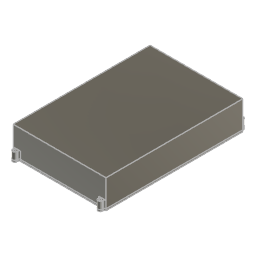
electronics holder (Autodesk Fusion 360 design; units mm, degrees)
part number: 2026-05-19-09-00-51-431
Autodesk Fusion 360 part; units mm, degrees
note: some values were not read from the file. Chosen so that the rebuilt part matches the saved one: which face or edge a step refers to; which pieces of a blend or face edit are solid. Set by a fixed rule: which sketch regions a step uses.
sketch "Sketch3" plane through (0, 0, 0) normal (0, 0, 1) x (1, 0, 0)
  line L0 (5, 13.5) -> (5, -13.5)
  line L1 (5, 13.5) -> (43, 13.5)
  line L2 (43, 13.5) -> (43, -13.5)
  line L3 (43, -13.5) -> (5, -13.5)
  line L4 (5, -13.5) -> (5, 13.5)
  line L5 (-5, -13.5) -> (-43, -13.5)
  line L6 (-43, -13.5) -> (-43, 13.5)
  line L7 (-43, 13.5) -> (-5, 13.5)
  line L8 (-5, 13.5) -> (-5, -13.5)
  line L9 (42.8, 30) -> (-42.8, 30)
  line L10 (42.8, 30) -> (-42.8, 30)
  line L11 (-42.8, 30) -> (-42.8, 86.5)
  line L12 (-42.8, 86.5) -> (42.8, 86.5)
  line L13 (42.8, 86.5) -> (42.8, 30)
  point P0 (5, 0)
  point P1 (0, 30)
  dimension "d5" = 27
  dimension "d6" = 38
  dimension "d7" = 27
  dimension "d8" = 38
  dimension "d9" = 27
  dimension "d10" = 85.6
  dimension "d11" = 56.5
  constraint midpoint L0 P0
  constraint vertical L0
  constraint horizontal L1
  constraint vertical L2
  constraint horizontal L3
  constraint vertical L4
  constraint horizontal L5
  constraint vertical L6
  constraint horizontal L7
  constraint vertical L8
  constraint midpoint L9 P1
  constraint horizontal L9
  constraint horizontal L10
  constraint vertical L11
  constraint horizontal L12
  constraint vertical L13
  measures "d5" distance of L0.start L0.end
  measures "d6" distance of L0.start L1.end
  measures "d7" distance of L0.start L0.end
  measures "d8" distance of L5.start L5.end
  measures "d9" distance of L5.start L7.end
  measures "d10" distance of L9.start L9.end
  measures "d11" distance of L9.start L12.end
extrude "Extrude2" add sketch "Sketch3" along normal blind 18 makes body 1 at (-30.3333, -4.5, 0) makes body 2 at (17.6667, -4.5, 0) makes body 3 at (14.2667, 48.8333, 0)
sketch "Sketch4" plane through (0, 0, 0) normal (0, 0, -1) x (1, 0, 0)
  line L0 (-42.8, -86.5) -> (42.8, -86.5)
  line L1 (42.8, -86.5) -> (42.8, -30)
  line L2 (42.8, -30) -> (-42.8, -30)
  line L3 (-42.8, -30) -> (-42.8, -86.5)
  line L4 (-52.8376, 24.1534) -> (52.8376, 24.1534)
  line L5 (52.8376, 24.1534) -> (52.8376, -104.1534)
  line L6 (52.8376, -104.1534) -> (-52.8376, -104.1534)
  line L7 (-52.8376, -104.1534) -> (-52.8376, 24.1534)
  line L8 (-52.8376, 24.1534) -> (52.8376, -104.1534) construction
  line L9 (52.8376, 24.1534) -> (-52.8376, -104.1534) construction
  line L10 (-76.82, -19.5117) -> (-61.32, -19.5117)
  line L11 (-61.32, -19.5117) -> (-61.32, 0.8883)
  line L12 (-61.32, 0.8883) -> (-76.82, 0.8883)
  line L13 (-76.82, 0.8883) -> (-76.82, -19.5117)
  point P0 (0, -40)
  dimension "d16" = 15.5
  dimension "d17" = 20.4
  constraint horizontal L4
  constraint perpendicular L4 L5
  constraint parallel L4 L6
  constraint parallel L5 L7
  constraint coincident L8 P0
  constraint coincident L9 P0
  constraint horizontal L10
  constraint vertical L11
  constraint horizontal L12
  constraint vertical L13
  measures "d16" distance of L10.start L10.end
  measures "d17" distance of L10.start L12.end
extrude "Extrude3" add sketch "Sketch4" along normal blind 2 separate body contours L0 L1 L2 L3 | L4 L5 L6 L7 makes body 4
extrude "Extrude4" add 1 faces at (52.8376, 18.6155, -0.6667) along direction (1, 0, 0) blind 20 on bodies 4 bodies 4
sketch "Sketch5" plane through (0, 0, 0) normal (0, 0, 1) x (-1, 0, 0)
  line L0 (-72.8376, -104.1534) -> (52.8376, -104.1534)
  line L1 (52.8376, -104.1534) -> (52.8376, 24.1534)
  line L2 (52.8376, 24.1534) -> (-72.8376, 24.1534)
  line L3 (-72.8376, 24.1534) -> (-72.8376, -104.1534)
  line L4 (-50, 10) -> (-65.5, 10)
  line L5 (-65.5, 10) -> (-65.5, -10.4)
  line L6 (-65.5, -10.4) -> (-50, -10.4)
  line L7 (-50, -10.4) -> (-50, 10)
  dimension "d20" = 15.5
  dimension "d21" = 20.4
  constraint horizontal L4
  constraint vertical L5
  constraint horizontal L6
  constraint vertical L7
  measures "d20" distance of L4.start L4.end
  measures "d21" distance of L4.start L6.end
extrude "Extrude5" add sketch "Sketch5" along normal blind 11 separate body contours L4 L5 L6 L7 makes body 5
extrude "Extrude6" add 1 faces at (72.8376, 18.6155, -0.6667) along direction (1, 0, 0) blind 2 on bodies 4 bodies 4
move_body "Move4" bodies 3 to x (1, 0, 0) y (0, 1, 0) z (0, 0, 1) at (0, -10, 0)
extrude "Extrude7" add 1 faces at (-10.2792, -24.1534, -0.6667) along direction (0, -1, 0) blind 60 on bodies 4 bodies 4
sketch "Sketch6" plane through (0, 0, 0) normal (0, 0, 1) x (-1, 0, 0)
  line L0 (-74.8376, -104.1534) -> (52.8376, -104.1534)
  line L1 (52.8376, -104.1534) -> (52.8376, 84.1534)
  line L2 (52.8376, 84.1534) -> (-74.8376, 84.1534)
  line L3 (-74.8376, 84.1534) -> (-74.8376, -104.1534)
  line L4 (-55.6225, 66.6829) -> (-1.6225, 66.6829)
  line L5 (-1.6225, 66.6829) -> (-1.6225, 7.1829)
  line L6 (-1.6225, 7.1829) -> (-55.6225, 7.1829)
  line L7 (-55.6225, 7.1829) -> (-55.6225, 66.6829)
  dimension "d28" = 54
  dimension "d29" = 59.5
  constraint horizontal L4
  constraint vertical L5
  constraint horizontal L6
  constraint vertical L7
  measures "d28" distance of L4.start L4.end
  measures "d29" distance of L4.start L6.end
extrude "Extrude8" add sketch "Sketch6" along normal blind 27.5 separate body contours L4 L5 L6 L7 makes body 6
move_body "Move5" bodies 6 to x (1, 0, 0) y (0, 1, 0) z (0, 0, 1) at (10, -13, 0)
copy_body "CopyPasteBodies5" bodies 6 makes body 7
move_body "Move7" bodies 7 to x (1, 0, 0) y (0, 1, 0) z (0, 0, 1) at (-55, 0, 0)
extrude "Extrude10" add 1 faces at (-10.2792, -84.1534, -0.6667) along direction (0, -1, 0) blind 5 on bodies 4 bodies 4
extrude "Extrude11" add 1 faces at (-10.2792, 104.1534, -0.6667) along direction (0, 1, 0) blind 30 on bodies 4 bodies 4
move_body "Move8" bodies 3 to x (0, -1, 0) y (1, 0, 0) z (0, 0, 1) at (-34.5302, 62.1751, 0)
move_body "Move9" bodies 1 to x (0, -1, 0) y (1, 0, 0) z (0, 0, 1) at (-32.393, -21.4631, 0)
move_body "Move10" bodies 2 to x (0, -1, 0) y (1, 0, 0) z (0, 0, 1) at (-31.9661, 67.0384, 0)
move_body "Move11" bodies 3 to x (1, 0, 0) y (0, 1, 0) z (0, 0, 1) at (2.2501, -30.8582, 0)
move_body "Move12" bodies 2 to x (1, 0, 0) y (0, 1, 0) z (0, 0, 1) at (-1.6072, 11.8933, 0)
move_body "Move13" bodies 1 to x (1, 0, 0) y (0, 1, 0) z (0, 0, 1) at (-0.6429, 5.143, 0)
extrude "Extrude12" cut 1 faces at (-10.2792, 134.1534, -0.6667) along direction (0, -1, 0) blind 15 on bodies 4 bodies 4
move_body "Move14" bodies 5 to x (0, -1, 0) y (1, 0, 0) z (0, 0, 1) at (60, 40, 0)
move_body "Move15" bodies 5 to x (1, 0, 0) y (0, 1, 0) z (0, 0, 1) at (-1.4153, 18.1129, 0)
copy_body "CopyPasteBodies6" bodies 5 makes body 8
move_body "Move16" bodies 8 to x (1, 0, 0) y (0, 1, 0) z (0, 0, 1) at (0, 20, 0)
copy_body "CopyPasteBodies7" bodies 8 makes body 9
move_body "Move17" bodies 9 to x (1, 0, 0) y (0, 1, 0) z (0, 0, 1) at (0, 20, 0)
sketch "Sketch7" plane through (0, 0, 0) normal (0, 0, 1) x (-1, 0, 0)
  line L0 (-74.8376, -119.1534) -> (52.8376, -119.1534)
  line L1 (52.8376, -119.1534) -> (52.8376, 89.1534)
  line L2 (52.8376, 89.1534) -> (-74.8376, 89.1534)
  line L3 (-74.8376, 89.1534) -> (-74.8376, -119.1534)
  line L4 (-68.8465, -53.2998) -> (-53.3465, -53.2998)
  line L5 (-53.3465, -53.2998) -> (-53.3465, -79.0998)
  line L6 (-53.3465, -79.0998) -> (-68.8465, -79.0998)
  line L7 (-68.8465, -79.0998) -> (-68.8465, -53.2998)
  dimension "d40" = 15.5
  dimension "d41" = 25.8
  constraint horizontal L4
  constraint vertical L5
  constraint horizontal L6
  constraint vertical L7
  measures "d40" distance of L4.start L4.end
  measures "d41" distance of L4.start L6.end
extrude "Extrude13" add sketch "Sketch7" along normal blind 3 separate body contours L4 L5 L6 L7 makes body 10
extrude "Extrude14" cut 1 faces at (-10.2792, 119.1534, -0.6667) along direction (0, -1, 0) blind 20 on bodies 4 bodies 4
move_body "Move18" bodies 3 to x (1, 0, 0) y (0, 1, 0) z (0, 0, 1) at (0, -5, 0)
sketch "Sketch8" plane through (0, 0, 0) normal (0, 0, 1) x (-1, 0, 0)
  line L0 (-74.8376, -99.1534) -> (52.8376, -99.1534)
  line L1 (52.8376, -99.1534) -> (52.8376, 89.1534)
  line L2 (52.8376, 89.1534) -> (-74.8376, 89.1534)
  line L3 (-74.8376, 89.1534) -> (-74.8376, -99.1534)
  line L4 (-74.8376, 89.1534) -> (-69.8376, 89.1534)
  line L5 (-69.8376, 89.1534) -> (-69.8376, 92.1534)
  circle A0 centre (-69.8376, 92.1534) radius 1.5
  line L6 (52.8376, 89.1534) -> (47.8376, 89.1534)
  line L7 (47.8376, 89.1534) -> (47.8376, 92.1534)
  circle A1 centre (47.8376, 92.1534) radius 1.5
  circle A2 centre (47.8376, 92.1534) radius 3
  circle A3 centre (-69.8376, 92.1534) radius 3
  line L8 (-69.8376, 92.1534) -> (-72.8376, 92.1534)
  line L9 (-72.8376, 92.1534) -> (-72.8376, 89.1533)
  line L10 (-66.8376, 92.1534) -> (-66.8376, 89.1534)
  line L11 (-66.8376, 89.1534) -> (-69.8376, 89.1534)
  line L12 (47.8376, 92.1534) -> (44.8376, 92.1534)
  line L13 (44.8376, 92.1534) -> (44.8376, 89.1534)
  line L14 (50.8376, 92.1534) -> (50.8376, 89.2905)
  line L15 (50.8376, 89.2905) -> (50.8376, 89.2)
  line L16 (50.8376, 89.2) -> (50.8398, 89.1534)
  line L17 (-11, 89.1534) -> (-11, -99.1534)
  line L18 (-11, -5) -> (37.3566, -5)
  circle A4 centre (-69.8376, -102.1534) radius 3
  line L19 (-69.8376, -102.1534) -> (-72.8376, -102.1534)
  line L20 (-72.8376, -102.1534) -> (-72.8376, -99.1533)
  line L21 (-74.8376, -99.1534) -> (-74.8376, 89.1534)
  line L22 (52.8376, -99.1534) -> (-74.8376, -99.1534)
  line L23 (-74.8376, -99.1534) -> (-69.8376, -99.1534)
  circle A5 centre (-69.8376, -102.1534) radius 1.5
  line L24 (-69.8376, -99.1534) -> (-69.8376, -102.1534)
  line L25 (-66.8376, -102.1534) -> (-66.8376, -99.1534)
  circle A6 centre (47.8376, -102.1534) radius 3
  circle A7 centre (47.8376, -102.1534) radius 1.5
  line L26 (52.8376, 89.1534) -> (52.8376, -99.1534)
  line L27 (52.8376, -99.1534) -> (47.8376, -99.1534)
  line L28 (50.8376, -102.1534) -> (50.8376, -99.2905)
  line L29 (47.8376, -102.1534) -> (44.8376, -102.1534)
  line L30 (44.8376, -102.1534) -> (44.8376, -99.1534)
  line L31 (47.8376, -99.1534) -> (47.8376, -102.1534)
  line L32 (50.8376, -99.2905) -> (50.8376, -99.2)
  line L33 (50.8398, -99.1534) -> (47.8376, -99.1534)
  line L34 (50.8376, -99.2) -> (50.8398, -99.1534)
  point P0 (50.8398, -99.1534)
  dimension "d46" = 5
  dimension "d47" = 3
  dimension "d48" = 3
  dimension "d49" = 5
  dimension "d50" = 3
  dimension "d51" = 3
  dimension "d52" = 6
  dimension "d53" = 6
  dimension "d54" = 90
  constraint coincident L2.end L3.start
  constraint perpendicular L3 L4
  constraint perpendicular L4 L5
  constraint coincident L5.end A0.centre
  constraint coincident L1.end L2.start
  constraint perpendicular L1 L6
  constraint perpendicular L6 L7
  constraint coincident L7.end A1.centre
  constraint concentric A1 A2
  constraint concentric A0 A3
  constraint coincident A3 L8.end
  constraint perpendicular L5 L8
  constraint coincident A3 L10.start
  constraint coincident L2 L10.end
  constraint tangent A3 L10
  constraint perpendicular L2 L10
  constraint coincident A2 L12.end
  constraint perpendicular L7 L12
  constraint coincident L2 L13.end
  constraint tangent A2 L13
  constraint coincident A2 L14.start
  constraint tangent A2 L14
  constraint perpendicular L6 L14
  constraint perpendicular L6 L15
  constraint coincident L6 L16.end
  constraint midpoint L2 L17.start
  constraint midpoint L0 L17.end
  constraint midpoint L17 L18.start
  constraint perpendicular L17 L18
  constraint symmetric L0.start L18 L2.end
  constraint symmetric L0.end L18 L1.end
  constraint symmetric L1.end L18 L0.end
  constraint symmetric L2.end L18 L0.start
  constraint symmetric L4.end L18 L23.end
  constraint symmetric L5.end L18 A4.centre
  constraint symmetric A0 L18 A5
  constraint symmetric L6.end L18 L27.end
  constraint symmetric L7.end L18 A6.centre
  constraint symmetric A1 L18 A7
  constraint symmetric A2 L18 A6
  constraint symmetric A3 L18 A4
  constraint symmetric L8.end L18 L19.end
  constraint symmetric L9.end L18 L20.end
  constraint symmetric L10.start L18 L25.start
  constraint symmetric L10.end L18 L25.end
  constraint symmetric L12.end L18 L29.end
  constraint symmetric L13.end L18 L30.end
  constraint symmetric L14.start L18 L28.start
  constraint symmetric L14.end L18 L28.end
  constraint symmetric L15.end L18 L32.end
  constraint symmetric L16.end L18 P0
  constraint coincident P0 L33.start
  measures "d46" distance of L2.end L4.end
  measures "d47" distance of L4.end L5.end
  measures "d48" diameter of A0
  measures "d49" distance of L1.end L6.end
  measures "d50" distance of L6.end L7.end
  measures "d51" diameter of A1
  measures "d52" diameter of A2
  measures "d53" diameter of A3
  measures "d54" angle of L8 L9
extrude "Extrude15" add sketch "Sketch8" against normal blind 2.4 contours L0 A4 L20 L22 L23 | L0 A4 L22 L25 | A4 L19 A5 L24 | A4 L19 A5 L24 | L2 L4 A3 L9 | L2 A3 L10 L11 | L5 A0 A3 L8 | L5 A0 A3 L8 | L0 L22 A6 L30 | L0 L22 A6 L27 L28 L32 L33 L34 | A6 A7 L29 L31 | A6 A7 L29 L31 | L2 A2 L13 | L2 L6 A2 L14 L15 L16 | L7 A1 A2 L12 | L7 A1 A2 L12 bodies 4
extrude "Extrude16" add 1 faces at (29.6125, 36.3845, -2) along direction (0, 0, -1) blind 0.4 on bodies 4 bodies 4
fillet "Fillet1" radius 2 1 edges at (72.8376, -89.1534, -1.2) on bodies 4
fillet "Fillet2" radius 2 1 edges at (66.8376, -89.1534, -1.2) on bodies 4
fillet "Fillet3" radius 2 6 edges at (-50.8376, -89.2, -1.2) (-44.8376, -89.1534, -1.2) (72.8376, 99.1534, -1.2) (66.8376, 99.1534, -1.2) (-50.8376, 99.2, -1.2) (-44.8376, 99.1534, -1.2) on bodies 4
fillet "Fillet4" radius 2 1 edges at (-50.8398, -89.1534, -1.2) on bodies 4
sketch "Sketch9" plane through (0, 0, 0) normal (0, 0, 1) x (-1, 0, 0)
  circle A0 centre (-69.8376, 92.1534) radius 1.5
  circle A1 centre (47.8376, -102.1534) radius 1.5
  circle A2 centre (47.8376, 92.1534) radius 1.5
  circle A3 centre (-69.8376, -102.1534) radius 1.5
  arc A4 (-72.8376, -101.1534) -> (-74.8376, -99.1534) centre (-74.8376, -101.1534) ccw
  line L0 (-72.8376, -101.1534) -> (-72.8376, -102.1534)
  arc A5 (-72.8376, -102.1534) -> (-66.8376, -102.1534) centre (-69.8376, -102.1534) ccw
  line L1 (-66.8376, -102.1534) -> (-66.8376, -101.1534)
  arc A6 (-64.8376, -99.1534) -> (-66.8376, -101.1534) centre (-64.8376, -101.1534) ccw
  line L2 (-64.8376, -99.1534) -> (42.8376, -99.1534)
  arc A7 (44.8376, -101.1534) -> (42.8376, -99.1534) centre (42.8376, -101.1534) ccw
  line L3 (44.8376, -101.1534) -> (44.8376, -102.1534)
  arc A8 (44.8376, -102.1534) -> (50.8376, -102.1534) centre (47.8376, -102.1534) ccw
  line L4 (50.8376, -102.1534) -> (50.8376, -99.2475)
  arc A9 (50.8398, -99.1534) -> (50.8376, -99.2475) centre (52.8376, -99.2475) ccw
  line L5 (50.8398, -99.1534) -> (52.8376, -99.1534)
  line L6 (52.8376, -99.1534) -> (52.8376, 89.1534)
  arc A10 (50.8376, 91.1534) -> (52.8376, 89.1534) centre (52.8376, 91.1534) ccw
  line L7 (50.8376, 91.1534) -> (50.8376, 92.1534)
  arc A11 (50.8376, 92.1534) -> (44.8376, 92.1534) centre (47.8376, 92.1534) ccw
  line L8 (44.8376, 92.1534) -> (44.8376, 91.1534)
  arc A12 (42.8376, 89.1534) -> (44.8376, 91.1534) centre (42.8376, 91.1534) ccw
  line L9 (42.8376, 89.1534) -> (-64.8376, 89.1534)
  arc A13 (-66.8376, 91.1534) -> (-64.8376, 89.1534) centre (-64.8376, 91.1534) ccw
  line L10 (-66.8376, 91.1534) -> (-66.8376, 92.1534)
  arc A14 (-66.8376, 92.1534) -> (-72.8376, 92.1534) centre (-69.8376, 92.1534) ccw
  line L11 (-72.8376, 92.1534) -> (-72.8376, 91.1534)
  arc A15 (-74.8376, 89.1534) -> (-72.8376, 91.1534) centre (-74.8376, 91.1534) ccw
  line L12 (-74.8376, 89.1534) -> (-74.8376, -99.1534)
  line L13 (52.8376, -99.1534) -> (52.8398, -99.1534)
  line L14 (50.8398, -101.1534) -> (50.8398, -103.2837)
  line L15 (52.8376, -99.1534) -> (52.8376, -102)
  line L16 (52.8376, -102) -> (50.8398, -102)
  arc A16 (52.8398, -99.1534) -> (50.8398, -101.1534) centre (52.8398, -101.1534) ccw
  line L17 (50.9, -102) -> (50.3077, -100.0414)
  line L18 (50.3077, -100.0414) -> (50.5604, -98.5323)
  line L19 (50.5604, -98.5323) -> (52.8398, -99.1534)
  dimension "d67" = 2
  constraint coincident L5.end L6.start
  constraint vertical L14
  constraint perpendicular L5 L15
  constraint coincident L14 L16.end
  constraint perpendicular L4 L16
  constraint tangent L13 A16
  constraint tangent L14 A16
  constraint coincident L16 L17.start
  measures "d67" radius of A16
extrude "Extrude17" add sketch "Sketch9" against normal blind 2.4 contours L4 A9 L5 L14 L17 L18 L19 | L4 A9 L5 A16 bodies 4
sketch "Sketch10" plane through (0, 0, 0) normal (0, 0, 1) x (-1, 0, 0)
  line L0 (50.8376, -101.801) -> (50.8376, -101.1534)
  arc A0 (52.8376, -99.1534) -> (50.8398, -101.1534) centre (52.8398, -101.1534) ccw
  line L1 (52.8376, -99.1534) -> (52.8376, 89.1534)
  arc A1 (50.8376, 91.1534) -> (52.8376, 89.1534) centre (52.8376, 91.1534) ccw
  line L2 (50.8376, 91.1534) -> (50.8376, 92.1534)
  arc A2 (50.8376, 92.1534) -> (44.8376, 92.1534) centre (47.8376, 92.1534) ccw
  line L3 (44.8376, 92.1534) -> (44.8376, 91.1534)
  arc A3 (42.8376, 89.1534) -> (44.8376, 91.1534) centre (42.8376, 91.1534) ccw
  line L4 (42.8376, 89.1534) -> (-64.8376, 89.1534)
  arc A4 (-66.8376, 91.1534) -> (-64.8376, 89.1534) centre (-64.8376, 91.1534) ccw
  line L5 (-66.8376, 91.1534) -> (-66.8376, 92.1534)
  arc A5 (-66.8376, 92.1534) -> (-72.8376, 92.1534) centre (-69.8376, 92.1534) ccw
  line L6 (-72.8376, 92.1534) -> (-72.8376, 91.1534)
  arc A6 (-74.8376, 89.1534) -> (-72.8376, 91.1534) centre (-74.8376, 91.1534) ccw
  line L7 (-74.8376, 89.1534) -> (-74.8376, -99.1534)
  arc A7 (-72.8376, -101.1534) -> (-74.8376, -99.1534) centre (-74.8376, -101.1534) ccw
  line L8 (-72.8376, -101.1534) -> (-72.8376, -102.1534)
  arc A8 (-72.8376, -102.1534) -> (-66.8376, -102.1534) centre (-69.8376, -102.1534) ccw
  line L9 (-66.8376, -102.1534) -> (-66.8376, -101.1534)
  arc A9 (-64.8376, -99.1534) -> (-66.8376, -101.1534) centre (-64.8376, -101.1534) ccw
  line L10 (-64.8376, -99.1534) -> (42.8376, -99.1534)
  arc A10 (44.8376, -101.1534) -> (42.8376, -99.1534) centre (42.8376, -101.1534) ccw
  line L11 (44.8376, -101.1534) -> (44.8376, -102.1534)
  arc A11 (44.8376, -102.1534) -> (50.8376, -102.1534) centre (47.8376, -102.1534) ccw
  line L12 (50.8376, -102.1534) -> (50.8376, -101.801)
  circle A12 centre (-69.8376, -102.1534) radius 1.5
  circle A13 centre (47.8376, 92.1534) radius 1.5
  circle A14 centre (47.8376, -102.1534) radius 1.5
  circle A15 centre (-69.8376, 92.1534) radius 1.5
  line L13 (-74.8376, -99.1534) -> (-74.8376, -97.1534)
  line L14 (-74.8376, -99.1534) -> (-72.8376, -99.1534)
  line L15 (-72.8376, -99.1534) -> (-73.0068, 88.2092)
  line L16 (-74.8376, 89.1534) -> (-74.8376, 87.1534)
  line L17 (-74.8376, 87.1534) -> (52.7862, 87.1534)
  line L18 (52.8376, 89.1534) -> (50.8376, 89.1534)
  line L19 (50.8376, 89.1534) -> (50.8376, -98)
  line L20 (52.8376, -99.1534) -> (52.8376, -97.1534)
  line L21 (52.8376, -97.1534) -> (-74.8376, -97.1534)
  line L22 (52.8376, -97.1534) -> (52.8376, 89.1534)
  line L23 (-74.8376, -97.1534) -> (52.8376, -97.1534)
  arc A16 (44.8376, -102.1534) -> (50.8376, -102.1534) centre (47.8376, -102.1534) ccw
  arc A17 (52.8376, -99.1534) -> (50.8398, -101.1534) centre (52.8398, -101.1534) ccw
  line L24 (50.8387, -101.801) -> (50.8387, -101.1534)
  line L25 (50.8376, -102.1534) -> (50.8387, -101.801)
  line L26 (44.8376, -102.1534) -> (44.8376, -101.1534)
  arc A18 (44.8376, -101.1534) -> (42.8376, -99.1534) centre (42.8376, -101.1534) ccw
  line L27 (-64.8376, -99.1534) -> (42.8376, -99.1534)
  arc A19 (-72.8376, -101.1534) -> (-74.8376, -99.1534) centre (-74.8376, -101.1534) ccw
  arc A20 (-72.8376, -102.1534) -> (-66.8376, -102.1534) centre (-69.8376, -102.1534) ccw
  line L28 (-72.8376, -102.1534) -> (-72.8376, -101.1534)
  line L29 (-66.8376, -102.1534) -> (-66.8376, -101.1534)
  arc A21 (-64.8376, -99.1534) -> (-66.8376, -101.1534) centre (-64.8376, -101.1534) ccw
  line L30 (47.8376, -99.1534) -> (47.8376, -102.1534)
  circle A22 centre (47.8376, -102.1534) radius 3
  line L31 (47.8376, -102.1534) -> (44.8376, -102.1534)
  circle A23 centre (47.8376, -102.1534) radius 1.5
  circle A24 centre (-69.8376, -102.1534) radius 3
  line L32 (-66.8376, -102.1534) -> (-66.8376, -99.1534)
  circle A25 centre (-69.8376, -102.1534) radius 1.5
  line L33 (-69.8376, -102.1534) -> (-72.8376, -102.1534)
  line L34 (-69.8376, -99.1534) -> (-69.8376, -102.1534)
  line L35 (-72.8376, -102.1534) -> (-72.8376, -99.1533)
  line L36 (50.8376, -102.1534) -> (50.8376, -101.1534)
  line L37 (50.8387, -101.1534) -> (52.8376, -99.1534)
  arc A26 (52.8376, -99.1534) -> (50.8376, -101.1534) centre (52.8376, -101.1534) ccw
  line L38 (52.8376, -99.1534) -> (-74.8376, -99.1534)
  line L39 (-74.8376, 89.1534) -> (52.8376, 89.1534)
  point P0 (-66.8376, -101.1534)
  point P1 (50.8376, -99.1534)
  dimension "d70" = 2
  dimension "d71" = 2
  dimension "d72" = 2
  dimension "d73" = 90
  dimension "d74" = 2
  dimension "d75" = 2
  dimension "d76" = 3
  dimension "d77" = 2
  constraint coincident L7.end A7.end
  constraint parallel L7 L13
  constraint perpendicular L7 L14
  constraint coincident A6.start L7.start
  constraint parallel L7 L16
  constraint coincident L1.end A1.end
  constraint tangent A1 L18
  constraint perpendicular L10 L19
  constraint coincident A0.start L1.start
  constraint coincident L1 L20.end
  constraint vertical L36
  constraint coincident A11.end L12.start
  constraint coincident L24.end L37.start
  constraint coincident P1 L36
  constraint tangent L36 A26
  measures "d70" distance of L7.end L13.end
  measures "d71" distance of L7.end L14.end
  measures "d72" distance of A6.start L16.end
  measures "d73" angle of L16 L17
  measures "d74" distance of L1.end L18.end
  measures "d75" distance of A0.start L20.end
  measures "d76" distance of A11.end P1
  measures "d77" radius of A26
extrude "Extrude18" add sketch "Sketch10" along normal blind 50 separate body contours L0 A0 L12 A17 L24 L25 A22 L36 A26 L38 | A11 A14 A16 L30 A22 L31 A23 | L1 L10 L15 L20 L21 L23 L27 L38 | A10 L11 L26 A18 A22 L38 | A14 L30 A22 L31 A23 | L1 L18 L19 L21 L22 L23 L39 | A1 L2 A2 L3 A3 L18 L39 | A9 A21 L32 L38 | L4 L7 L16 L17 L19 L39 | L7 L15 L17 L21 L23 | L7 L13 L14 L15 L21 L23 L38 | L9 L29 A24 L32 L38 | A7 L14 A19 L35 L38 | L8 L28 A24 L35 L38 | A8 A12 A20 A24 A25 L33 L34 | A12 A24 A25 L33 L34 | A4 L5 A5 L6 A6 L39 makes body 11
extrude "Extrude19" cut 1 faces at (-47.4321, -89.1566, 50) along direction (0, 0, -1) blind 40 on bodies 11 bodies 11
extrude "Extrude20" add sketch "Sketch10" along normal blind 30 separate body contours L1 L10 L15 L20 L21 L23 L27 L38 | L1 L18 L19 L21 L22 L23 L39 | L4 L7 L16 L17 L19 L39 | L7 L15 L17 L21 L23 | L7 L13 L14 L15 L21 L23 L38 makes body 12
combine "Combine1" operation add target body 12 tool bodies 11
move_face "OffsetFaces1" offset 0.168 1 faces at (72.8949, 35.7178, 10) on bodies 12
extrude "Extrude21" add 1 faces at (-7.0013, 97.82, 30) along direction (0, 0, 1) blind 5 on bodies 12 bodies 12
sketch "Sketch11" plane through (0, 0, 35) normal (0, 0, 1) x (-1, 0, 0)
  line L0 (50.8376, -97.1534) -> (-72.6714, -97.1534)
  line L1 (-72.6714, -97.1534) -> (-72.8379, 87.1534)
  line L2 (-72.8379, 87.1534) -> (50.8376, 87.1534)
  line L3 (50.8376, 87.1534) -> (50.8376, -97.1534)
  line L4 (-74.8376, 89.1534) -> (-74.8376, -99.1534)
  line L5 (-74.8376, -99.1534) -> (52.8376, -99.1534)
  line L6 (52.8376, -99.1534) -> (52.8376, 89.1534)
  line L7 (52.8376, 89.1534) -> (-74.8376, 89.1534)
  line L8 (-74.8376, 89.1534) -> (52.8376, 89.1534)
  line L9 (52.8376, 89.1534) -> (52.8376, -99.1534)
  line L10 (52.8376, -99.1534) -> (-74.8376, -99.1534)
  line L11 (-74.8376, -99.1534) -> (-74.8376, 89.1534)
  constraint horizontal L8
  constraint vertical L9
  constraint horizontal L10
  constraint vertical L11
  constraint coincident L5.end L6.start
  constraint coincident L4.start L7.end
extrude "Extrude22" add sketch "Sketch11" along normal blind 2 contours L0 L1 L2 L3 | L4 L5 L6 L7 L8 L9 L10 L11 bodies 12
sketch "Sketch12" plane through (74.8376, 0, 0) normal (1, 0, 0) x (0, 1, 0)
  line L0 (99.1534, 10) -> (99.1534, 35)
  line L1 (99.1534, 35) -> (99.1534, 37)
  line L2 (99.1534, 37) -> (-89.1534, 37)
  line L3 (-89.1534, 37) -> (-89.1534, 10)
  line L4 (-89.1534, 10) -> (-89.1534, 0)
  line L5 (-89.1534, 0) -> (99.1534, 0)
  line L6 (99.1534, 0) -> (99.1534, 10)
  line L7 (5, 37) -> (5, -2.4)
  line L8 (5, 17.3) -> (5, 26.825)
  line L9 (5, 17.3) -> (5, 7.775)
  line L10 (5, 7.775) -> (14.525, 7.775)
  line L11 (14.525, 7.775) -> (14.525, 26.825)
  line L12 (14.525, 26.825) -> (-4.525, 26.825)
  line L13 (-4.525, 26.825) -> (-4.525, 7.775)
  line L14 (-4.525, 7.775) -> (14.525, 7.775)
  point P0 (5, 26.1052)
  dimension "d90" = 9.525
  dimension "d91" = 9.525
  dimension "d92" = 9.525
  dimension "d93" = 19.05
  dimension "d94" = 19.05
  dimension "d95" = 19.05
  constraint midpoint L2 L7.start
  constraint perpendicular L5 L7
  constraint midpoint L7 L8.start
  constraint parallel L7 L8
  constraint parallel L7 L9
  constraint perpendicular L7 L10
  constraint perpendicular L10 L11
  constraint perpendicular L7 L12
  constraint perpendicular L12 L13
  measures "d90" distance of L8.start L8.end
  measures "d91" distance of L8.start L9.end
  measures "d92" distance of L9.end L10.end
  measures "d93" distance of L10.end L11.end
  measures "d94" distance of L11.end L12.end
  measures "d95" distance of L12.end L13.end
sketch "Sketch13" plane through (0, 0, 37) normal (0, 0, 1) x (-1, 0, 0)
  line L0 (-74.8376, -99.1534) -> (52.8376, -99.1534)
  line L1 (52.8376, -99.1534) -> (52.8376, 89.1534)
  line L2 (52.8376, 89.1534) -> (-74.8376, 89.1534)
  line L3 (-74.8376, 89.1534) -> (-74.8376, -99.1534)
  circle A0 centre (154.6142, -13.5152) radius 4.572
  circle A1 centre (154.6142, -13.5152) radius 5
  dimension "d96" = 9.144
  dimension "d97" = 10
  constraint concentric A0 A1
  measures "d96" diameter of A0
  measures "d97" diameter of A1
combine "Combine2" [no effect]
sketch "Sketch14" plane through (0, 0, 0) normal (1, 0, 0) x (0, 1, 0)
  circle A0 centre (-180, 10) radius 4
  circle A1 centre (-180, 10) radius 7.5
  dimension "d102" = 8
  dimension "d103" = 15
  constraint concentric A0 A1
  measures "d102" diameter of A0
  measures "d103" diameter of A1
extrude "Extrude25" add sketch "Sketch14" along normal blind 2 separate body makes body 13
sketch "Sketch15" plane through (2, 0, 0) normal (1, 0, 0) x (0, 1, 0)
  circle A0 centre (-180, 10) radius 4
  circle A1 centre (-180, 10) radius 7.5
  circle A2 centre (-180, 10) radius 5
  circle A3 centre (-180, 10) radius 10
  dimension "d106" = 10
  dimension "d107" = 20
  constraint concentric A0 A2
  constraint concentric A0 A3
  measures "d106" diameter of A2
  measures "d107" diameter of A3
extrude "Extrude26" add sketch "Sketch15" along normal blind 3 contours A1 | A3 bodies 13
extrude "Extrude27" add 1 faces at (2, -170.8985, 9.1306) along direction (-1, 0, 0) blind 2 on bodies 13 bodies 13
sketch "Sketch16" plane through (0, 0, 0) normal (-1, 0, 0) x (0, -1, 0)
  circle A0 centre (180, 10) radius 10
  circle A1 centre (180, 10) radius 4
  line L0 (179.7063, 13.9892) -> (179.7063, 20.371)
  line L1 (179.7063, 20.371) -> (180.1406, 20.371)
  line L2 (180.1406, 20.371) -> (180.1406, 13.9335)
  line L3 (180.1406, 13.9335) -> (179.7063, 13.9892)
  dimension "d112" = 90
  constraint coincident A1 L0.start
  constraint vertical L0
  constraint perpendicular L0 L1
  measures "d112" angle of L1 L2
extrude "Extrude28" cut sketch "Sketch16" against normal blind 30 contours A0 A1 L0 L2 picked at (180.0924, 15.9988) bodies 13
sketch "Sketch17" plane through (0, 0, 0) normal (-1, 0, 0) x (0, -1, 0)
  line L0 (179.7063, 13.9892) -> (179.7063, 19.9957)
  arc A0 (179.7063, 19.9957) -> (180.1406, 19.999) centre (180, 10) ccw
  line L1 (180.1406, 19.999) -> (180.1406, 13.9975)
  arc A1 (179.7063, 13.9892) -> (180.1406, 13.9975) centre (180, 10) ccw
  line L2 (173, 2) -> (189.1864, 2)
  line L3 (189.1864, 2) -> (189.1864, -1.6073)
  line L4 (189.1864, -1.6073) -> (173, -1.6073)
  line L5 (173, -1.6073) -> (173, 2)
  line L6 (179, 6.5) -> (179.5, 6.5)
  line L7 (179.5, 6.5) -> (179.5, 4)
  line L8 (179.5, 4) -> (179, 4)
  line L9 (179, 4) -> (179, 6.5)
  constraint horizontal L2
  constraint vertical L3
  constraint horizontal L4
  constraint vertical L5
  constraint horizontal L6
  constraint vertical L7
  constraint horizontal L8
  constraint vertical L9
extrude "Extrude29" cut sketch "Sketch17" against normal blind 34 contours A0 L2 bodies 13
extrude "Extrude30" cut sketch "Sketch17" against normal blind 30 contours A1 L7 L8 L9 bodies 13
extrude "Extrude31" add 1 faces at (5, -179.8333, 2.6667) along direction (1, 0, 0) blind 1 on bodies 13 bodies 13
extrude "Extrude32" add 1 faces at (6, -179.8333, 2.6667) along direction (1, 0, 0) blind 1 on bodies 13 bodies 13
sketch "Sketch18" plane through (7, 0, 0) normal (1, 0, 0) x (0, 1, 0)
  line L0 (-179, 5.101) -> (-179, 4)
  line L1 (-179, 4) -> (-179.5, 4)
  line L2 (-179.5, 4) -> (-179.5, 5.0251)
  arc A0 (-180.1406, 14.998) -> (-179.5, 5.0251) centre (-180, 10) ccw
  line L3 (-180.1406, 14.998) -> (-180.1406, 19.999)
  arc A1 (-180.1406, 19.999) -> (-186, 2) centre (-180, 10) ccw
  line L4 (-186, 2) -> (-174, 2)
  arc A2 (-174, 2) -> (-179.7063, 19.9957) centre (-180, 10) ccw
  line L5 (-179.7063, 19.9957) -> (-179.7063, 14.9914)
  arc A3 (-179, 5.101) -> (-179.7063, 14.9914) centre (-180, 10) ccw
  circle A4 centre (-180, 10) radius 13.5
  circle A5 centre (-180, 10) radius 7.4993
  dimension "d123" = 27
  constraint concentric A0 A4
  constraint concentric A0 A5
  measures "d123" diameter of A4
extrude "Extrude33" add sketch "Sketch18" against normal blind 1 bodies 13
extrude "Extrude34" add 1 faces at (6, -179.6637, 0.1792) along direction (-1, 0, 0) blind 1 separate body on bodies 13 makes body 14
move_body "Move19" bodies 14 to x (1, 0, 0) y (0, 1, 0) z (0, 0, 1) at (-5, 0, 0)
sketch "Sketch19" plane through (0, 0, 0) normal (-1, 0, 0) x (0, -1, 0)
  line L0 (179, 4) -> (179, 6.127)
  arc A0 (179.7063, 13.9892) -> (179, 6.127) centre (180, 10) ccw
  line L1 (179.7063, 13.9892) -> (179.7063, 19.9957)
  arc A1 (179.7063, 19.9957) -> (174, 2) centre (180, 10) ccw
  line L2 (174, 2) -> (186, 2)
  arc A2 (186, 2) -> (180.1406, 19.999) centre (180, 10) ccw
  line L3 (180.1406, 19.999) -> (180.1406, 13.9975)
  arc A3 (179.5, 6.0314) -> (180.1406, 13.9975) centre (180, 10) ccw
  line L4 (179.5, 6.0314) -> (179.5, 4)
  line L5 (179.5, 4) -> (179, 4)
  line L6 (179.8303, 24.6232) -> (194.7877, 24.6232)
  line L7 (194.7877, 24.6232) -> (194.7877, -6.5435)
  line L8 (194.7877, -6.5435) -> (179.8303, -6.5435)
  line L9 (179.8303, -6.5435) -> (179.8303, 24.6232)
  constraint horizontal L6
  constraint vertical L7
  constraint horizontal L8
  constraint vertical L9
extrude "Extrude35" cut sketch "Sketch19" against normal blind 34 contours L2 A2 L3 A3 L6 L7 L8 L9 | L2 A2 L3 A3 L9 bodies 13 14
combine "Combine3" operation add target body 14 tool bodies 13
hidden bodies 14
equation "d84 = -1.832 mm + 2 mm"
equation "d90 = ( 19.05 / 2 ) * 1 mm"
equation "d91 = ( 19.05 / 2 ) * 1 mm"
equation "d92 = ( 19.05 / 2 ) * 1 mm"
named bodies: "electronics holder bottom casing", "electronics holder top casing"
